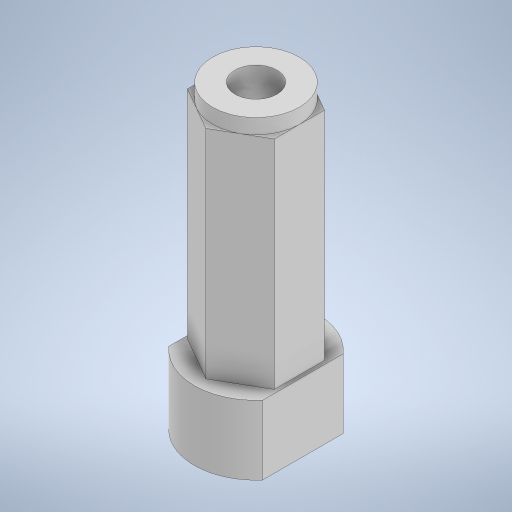
# Autodesk Inventor part: motor_to_mecanum_connector
Saved by Autodesk Inventor 2023.2 (Build 272271030, 271C)
## iProperties
Created: 2023-03-29
Part Number: motor_to_mecanum_connector
Material: Generic
Document SubType Name: Modeling
Designer: kao91
Density: 1 g/cm^3
Appearance: Default
Author: kao91
Autodesk Inventor part; units mm, degrees
ref_plane "YZ Plane" through (0, 0, 0) normal (1, 0, 0) x (0, 1, 0)
ref_plane "XZ Plane" through (0, 0, 0) normal (0, 1, 0) x (-1, 0, 0)
ref_plane "XY Plane" through (0, 0, 0) normal (0, 0, 1) x (1, 0, 0)
sketch "Sketch1" plane through (0, 0, 0) normal (0, 1, 0) x (-1, 0, 0)
  circle A0 centre (0, 0) radius 4.55
  line L0 (3.45, 4.55) -> (3.45, -4.55)
  line L1 (3.45, -4.55) -> (-3.45, -4.55)
  line L2 (-3.45, -4.55) -> (-3.45, 4.55)
  line L3 (-3.45, 4.55) -> (3.45, 4.55)
  line L4 (3.45, 4.55) -> (-3.45, -4.55) construction
  line L5 (3.45, -4.55) -> (-3.45, 4.55) construction
  circle A1 centre (0, 0) radius 2.8
  line L6 (1.95, 2.8) -> (1.95, -2.8)
  line L7 (1.95, -2.8) -> (-1.95, -2.8)
  line L8 (-1.95, -2.8) -> (-1.95, 2.8)
  line L9 (-1.95, 2.8) -> (1.95, 2.8)
  line L10 (1.95, 2.8) -> (-1.95, -2.8) construction
  line L11 (1.95, -2.8) -> (-1.95, 2.8) construction
  point P0 (-3.45, 2.9665)
  point P1 (-3.45, -2.9665)
  point P2 (3.45, -2.9665)
  point P3 (3.45, 2.9665)
  point P4 (-1.95, -2.0094)
  point P5 (-1.95, 2.0094)
  point P6 (1.95, 2.0094)
  point P7 (1.95, -2.0094)
  dimension "d0" = 9.1
  dimension "d1" = 9.1
  dimension "d2" = 6.9
  dimension "d3" = 5.6
  dimension "d4" = 5.6
  dimension "d5" = 3.9
  constraints: 24 end point, 4 midpoint, 4 parallel, 2 centre point, 2 coincident, 2 perpendicular, 2 vertical
  measures "d0" diameter of A0
  measures "d1" distance of L0.start L0.end
  measures "d2" distance of L0.end L1.end
  measures "d3" diameter of A1
  measures "d4" distance of L6.start L6.end
  measures "d5" distance of L6.end L7.end
extrude "Extrusion1" add sketch "Sketch1" against normal blind 5.1 contours L0 A0 L2 | A1 L6 | A1 L9 L6 | L6 L7 A1 | A1 L8 L9 | L7 L8 A1 | L8 A1
sketch "Sketch2" plane through (0, 0, 0) normal (0, 1, 0) x (1, 0, 0)
  line L0 (-3.2, 1.8475) -> (0, 3.695)
  line L1 (0, 3.695) -> (3.2, 1.8475)
  line L2 (3.2, 1.8475) -> (3.2, -1.8475)
  line L3 (3.2, -1.8475) -> (0, -3.695)
  line L4 (0, -3.695) -> (-3.2, -1.8475)
  line L5 (-3.2, -1.8475) -> (-3.2, 1.8475)
  circle A0 centre (0, 0) radius 1.55
  dimension "d8" = 6.4
  dimension "d9" = 6.4
  dimension "d10" = 3.1
  constraints: 12 end point, 2 coincident, 1 centre point, 13 other
  measures "d8" distance between parallel lines of L2 L5
  measures "d9" distance between parallel lines of L3 L0
  measures "d10" diameter of A0
extrude "Extrusion2" add sketch "Sketch2" along normal blind 16
sketch "Sketch3" plane through (0, 0, 0) normal (0, -1, 0) x (1, 0, 0)
  point P0 (0, 0)
sketch "Sketch4" plane through (0, 0, 0) normal (0, -1, 0) x (1, 0, 0)
  point P0 (0, 0)
sketch "Sketch5" plane through (0, 0, 0) normal (0, -1, 0) x (1, 0, 0)
  circle A0 centre (0, 0) radius 1.55 projected
  line L0 (1.95, -2.0094) -> (1.95, 2.0094) projected
  arc A1 (1.95, 2.0094) -> (-1.95, 2.0094) centre (0, 0) ccw projected
  line L1 (-1.95, 2.0094) -> (-1.95, -2.0094) projected
  arc A2 (-1.95, -2.0094) -> (1.95, -2.0094) centre (0, 0) ccw projected
extrude "Extrusion3" cut sketch "Sketch5" against normal blind 3
sketch "Sketch6" plane through (0, 16, 0) normal (0, 1, 0) x (1, 0, 0)
  circle A0 centre (0, 0) radius 3.2
  circle A1 centre (0, 0) radius 1.55
  constraints: 2 centre point, 2 coincident
extrude "Extrusion4" add sketch "Sketch6" along normal blind 1.1
body "Solid1"
